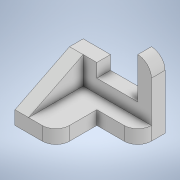
# Autodesk Inventor part: 零件5
Saved by Autodesk Inventor 2020 (Build 240168000, 168)
## iProperties
Created: 2020-09-19
Part Number: 零件5
Material: 一般
Document SubType Name: Modeling
Designer: User
Density: 1 g/cm^3
Appearance: 預設
Author: User
Autodesk Inventor part; units mm, degrees
ref_plane "YZ Plane" through (0, 0, 0) normal (1, 0, 0) x (0, 1, 0)
ref_plane "XZ Plane" through (0, 0, 0) normal (0, 1, 0) x (-1, 0, 0)
ref_plane "XY Plane" through (0, 0, 0) normal (0, 0, 1) x (1, 0, 0)
sketch "草圖1" plane through (0, 0, 0) normal (0, 0, 1) x (1, 0, 0)
  line L0 (0, 0) -> (60, 0)
  line L1 (60, 0) -> (60, 10)
  line L2 (60, 10) -> (0, 10)
  line L3 (0, 10) -> (0, 0)
  line L4 (60, 10) -> (60, 50)
  line L5 (60, 50) -> (50, 50)
  line L6 (50, 50) -> (50, 20)
  line L7 (50, 20) -> (20, 20)
  line L8 (20, 20) -> (20, 30)
  line L9 (20, 30) -> (10, 30)
  line L10 (10, 30) -> (10, 10)
  line L11 (30, 10) -> (30, 0)
  dimension "d0" = 60
  dimension "d1" = 10
  dimension "d2" = 40
  dimension "d3" = 10
  dimension "d4" = 30
  dimension "d5" = 30
  dimension "d6" = 10
  dimension "d7" = 10
  constraints: 24 end point, 7 perpendicular, 2 midpoint, 2 parallel, 1 horizontal, 1 point on line, 1 vertical
  measures "d0" distance of L2.end L1.end
  measures "d1" distance of L1.end L0.end
  measures "d2" distance of L1.end L4.end
  measures "d3" distance of L4.end L5.end
  measures "d4" distance of L5.end L6.end
  measures "d5" distance of L6.end L7.end
  measures "d6" distance of L7.end L8.end
  measures "d7" distance of L8.end L9.end
extrude "擠出1" add sketch "草圖1" along normal blind 20 contours L11 L2 L1 L0
extrude "擠出2" add sketch "草圖1" along normal blind 10 contours L2 L10 L9 L8 L7 L6 L5 L4
extrude "擠出3" add sketch "草圖1" along normal blind 50 contours L3 L2 L11 L0
fillet "圓角1" radius 10 3 edges at (30, 5, 50) (60, 5, 20) (60, 50, 5)
sketch "草圖2" plane through (0, 0, 0) normal (-1, 0, 0) x (0, 0, 1)
  line L0 (0, 10) -> (10, 10) projected
  line L1 (0, 30) -> (0, 10) projected
  line L2 (0, 10) -> (0, 30)
  line L3 (10, 20) -> (10, 30) projected
  line L4 (0, 30) -> (10, 30)
  line L5 (10, 30) -> (50, 10)
  line L6 (50, 10) -> (0, 10)
  point P0 (0, 0)
  dimension "d15" = 20
  constraints: 8 end point, 1 collinear, 1 parallel, 1 perpendicular
  measures "d15" distance of L0.start L1.start
extrude "擠出4" add sketch "草圖2" against normal blind 10
